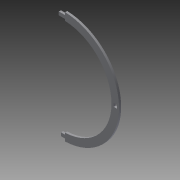
# Autodesk Inventor part: TopfemaleHoopSection_v2
Saved by Autodesk Inventor 2013 (Build 170138000, 138)
## iProperties
Created: 2013-01-17
Part Number: TopfemaleHoopSection_v2
Material: Generic
Document SubType Name: Modeling
Designer: twsass
Density: 1 g/cm^3
Author: twsass
Autodesk Inventor part; units mm, degrees
ref_plane "YZ Plane" through (0, 0, 0) normal (1, 0, 0) x (0, 1, 0)
ref_plane "XZ Plane" through (0, 0, 0) normal (0, 1, 0) x (-1, 0, 0)
ref_plane "XY Plane" through (0, 0, 0) normal (0, 0, 1) x (1, 0, 0)
sketch "Sketch1" plane through (0, 0, 0) normal (0, 0, 1) x (1, 0, 0)
  circle A0 centre (0, 0) radius 146.05
  circle A1 centre (0, 0) radius 168.91
  line L0 (6.35, -145.9119) -> (6.35, -168.7906)
  circle A2 centre (-157.48, 0) radius 3.175
  line L1 (6.35, -145.9119) -> (6.35, -150.9919)
  line L2 (6.35, -150.9919) -> (-6.35, -150.9919)
  line L3 (-6.35, -150.9919) -> (-6.35, -161.1519)
  line L4 (-6.35, -161.1519) -> (6.35, -161.1519)
  line L5 (6.35, -150.9919) -> (6.35, -161.1519)
  line L6 (157.48, 0) -> (157.48, 5.08)
  line L7 (157.48, 5.08) -> (162.2425, 5.08)
  line L8 (162.2425, 5.08) -> (162.2425, -5.08)
  line L9 (162.2425, -5.08) -> (152.7175, -5.08)
  line L10 (152.7175, -5.08) -> (152.7175, 5.08)
  line L11 (152.7175, 5.08) -> (157.48, 5.08)
  line L12 (6.35, 145.9119) -> (6.35, 168.7906)
  line L13 (0, 0) -> (0, 200.5264) construction
  line L14 (6.35, 145.9119) -> (6.35, 150.9919) construction
  line L15 (6.35, 150.9919) -> (-12.7, 150.9919)
  line L16 (-12.7, 150.9919) -> (-12.7, 161.1519)
  line L17 (-12.7, 161.1519) -> (6.35, 161.1519)
  line L18 (0, -146.05) -> (0, 0) construction
  point P0 (0.0447, 168.91)
  point P1 (6.3947, 145.9099)
  dimension "d51" = 292.1
  dimension "d52" = 337.82
  dimension "d58" = 5.08
  dimension "d59" = 12.7
  dimension "d60" = 10.16
  dimension "d63" = 5.08
  dimension "d64" = 4.7625
  dimension "d65" = 10.16
  dimension "d66" = 9.525
  dimension "d67" = 157.48
  dimension "d72" = 6.35
  dimension "d73" = 5.08
  dimension "d75" = 19.05
  dimension "d76" = 10.16
  dimension "d77" = 6.35
  constraints: 38 end point, 7 point on circle, 5 parallel, 5 perpendicular, 3 centre point, 2 collinear, 2 point on line, 1 coincident, 1 vertical
  measures "d51" diameter of A0
  measures "d52" diameter of A1
  measures "d58" distance of L0.start L1.end
  measures "d59" distance of L1.end L2.end
  measures "d60" distance of L2.end L3.end
  measures "d63" distance of L6.start L6.end
  measures "d64" distance of L6.end L7.end
  measures "d65" distance of L7.end L8.end
  measures "d66" distance of L8.end L9.end
  measures "d67" distance of A0.centre L6.start
  measures "d72" distance between parallel lines of L12 L13
  measures "d73" distance of L12.start L14.end
  measures "d75" distance of L14.end L15.end
  measures "d76" distance of L15.end L16.end
  measures "d77" distance between parallel lines of L18 L1
extrude "Extrusion13" add sketch "Sketch1" along normal blind 6.35 contours A0 L12 A1 L0 | L15 L16 L17 L12 | L0 L4 L3 L2
body "Solid6"
